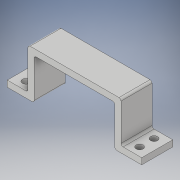
# Autodesk Inventor part: servoPlateConnection
Saved by Autodesk Inventor 2017 (Build 210142000, 142)
## iProperties
Created: 2017-04-22
Part Number: servoPlateConnection
Material: Generic
Document SubType Name: Modeling
Designer: s4461999
Density: 1 g/cm^3
Appearance: Default
Author: s4461999
Autodesk Inventor part; units mm, degrees
ref_plane "YZ Plane" through (0, 0, 0) normal (1, 0, 0) x (0, 1, 0)
ref_plane "XZ Plane" through (0, 0, 0) normal (0, 1, 0) x (-1, 0, 0)
ref_plane "XY Plane" through (0, 0, 0) normal (0, 0, 1) x (1, 0, 0)
sketch "Sketch1" plane through (0, 0, 0) normal (0, 0, 1) x (1, 0, 0)
  line L0 (0, 0) -> (12, 0)
  line L1 (13, 1) -> (13, 18.7)
  line L2 (14, 19.7) -> (51, 19.7)
  line L3 (52, 18.7) -> (52, 1)
  line L4 (53, 0) -> (65, 0)
  line L5 (65, 0) -> (65, 3)
  line L6 (65, 3) -> (56, 3)
  line L7 (55, 4) -> (55, 21.7)
  line L8 (54, 22.7) -> (11, 22.7)
  line L9 (10, 21.7) -> (10, 4)
  line L10 (9, 3) -> (0, 3)
  line L11 (0, 3) -> (0, 0)
  arc A0 (11, 22.7) -> (10, 21.7) centre (11, 21.7) ccw
  arc A1 (14, 19.7) -> (13, 18.7) centre (14, 18.7) ccw
  arc A2 (9, 3) -> (10, 4) centre (9, 4) ccw
  arc A3 (12, 0) -> (13, 1) centre (12, 1) ccw
  arc A4 (55, 4) -> (56, 3) centre (56, 4) ccw
  arc A5 (55, 21.7) -> (54, 22.7) centre (54, 21.7) ccw
  arc A6 (52, 18.7) -> (51, 19.7) centre (51, 18.7) ccw
  arc A7 (52, 1) -> (53, 0) centre (53, 1) ccw
  point P0 (52, 0)
  dimension "d0" = 3
  dimension "d1" = 3
  dimension "d2" = 3
  dimension "d3" = 3
  dimension "d4" = 3
  dimension "d5" = 19.7
  dimension "d6" = 39
  dimension "d7" = 10
  dimension "d8" = 10
  dimension "d9" = 1
  dimension "d10" = 1
  constraints: 24 end point, 16 point on circle, 16 tangent, 9 perpendicular, 8 centre point, 6 equal radius, 4 point on line, 1 horizontal, 1 vertical
  measures "d0" distance between parallel lines of L8 L2
  measures "d1" distance between parallel lines of L3 L7
  measures "d2" distance between parallel lines of L9 L1
  measures "d3" distance between parallel lines of L10 L0
  measures "d4" distance between parallel lines of L6 L4
  measures "d5" distance between parallel lines of L0 L2
  measures "d6" distance between parallel lines of L3 L1
  measures "d7" distance between parallel lines of L11 L9
  measures "d8" distance between parallel lines of L5 L7
  measures "d9" radius of A0
  measures "d10" radius of A5
extrude "Extrusion1" add sketch "Sketch1" along normal blind 15
sketch "Sketch2" plane through (0, 3, 0) normal (0, 1, 0) x (1, 0, 0)
  line L0 (65, 0) -> (56, 0) projected
  line L1 (65, -15) -> (56, -15) projected
  line L2 (9, 0) -> (0, 0) projected
  line L3 (9, -15) -> (0, -15) projected
  line L4 (65, 0) -> (65, -15) projected
  line L5 (0, 0) -> (0, -15) projected
  point P0 (60, -4)
  point P1 (60, -11)
  point P2 (5, -11)
  point P3 (5, -4)
  dimension "d13" = 4
  dimension "d14" = 4
  dimension "d15" = 4
  dimension "d16" = 4
  dimension "d17" = 5
  dimension "d18" = 5
  dimension "d19" = 5
  dimension "d20" = 5
  measures "d13" distance from line of point (60, -4) L0
  measures "d14" distance from line of L1 point (60, -11)
  measures "d15" distance from line of point (5, -4) L2
  measures "d16" distance from line of L3 point (5, -11)
  measures "d17" distance from line of L4 point (60, -11)
  measures "d18" distance from line of L4 point (60, -4)
  measures "d19" distance from line of point (5, -4) L5
  measures "d20" distance from line of L5 point (5, -11)
hole "Hole1" at (60, 3, 4) at (60, 3, 11) at (5, 3, 11) at (5, 3, 4) direction (0, -1, 0) diameter 3.4 end through all
body "Solid1"
